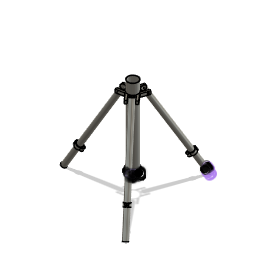
OpenTripod (Autodesk Fusion 360 design; units mm, degrees)
Autodesk Fusion 360 part; units mm, degrees
sketch "Sketch4" plane through (0, 0, 0) normal (0, 1, 0) x (1, 0, 0)
  circle A0 centre (0, 0) radius 25
  circle A1 centre (0, 0) radius 23
  dimension "d26" = 50
  dimension "d27" = 46
  constraint coincident A0.centre A1.centre
  constraint concentric A0 A1
  measures "d26" diameter of A0
  measures "d27" diameter of A1
extrude "Extrude6" add sketch "Sketch4" along normal blind 1000 makes body 1
sketch "Sketch1" plane through (0, 0, 0) normal (0, 1, 0) x (1, 0, 0)
  circle A0 centre (0, 0) radius 50
  circle A1 centre (0, 0) radius 47.5
  dimension "d1" = 100
  dimension "d2" = 95
  constraint coincident A0.centre A1.centre
  constraint concentric A0 A1
  measures "d1" diameter of A0
  measures "d2" diameter of A1
extrude "Extrude1" add sketch "Sketch1" along normal blind 800 separate body makes body 2
sketch "Sketch2" plane through (0, 800, 0) normal (0, 1, 0) x (-1, 0, 0)
  circle A0 centre (0, 0) radius 47.5
  circle A1 centre (0, 0) radius 50
  circle A2 centre (0, 0) radius 51
  circle A3 centre (0, 0) radius 60
  line L0 (0, 0) -> (-51, 0) construction
  line L1 (-51, 0) -> (-60, 0)
  line L2 (0, 0) -> (59.0885, 10.4189) construction
  line L3 (0, 0) -> (60, 0) construction
  line L4 (59.0885, 10.4189) -> (93.5567, 16.4966) construction
  circle A4 centre (93.5567, 16.4966) radius 25
  line L5 (93.5567, 16.4966) -> (89.2155, 41.1168) construction
  line L6 (89.2155, 41.1168) -> (88.3473, 46.0408) construction
  line L7 (88.3473, 46.0408) -> (45.9627, 38.5673)
  line L8 (88.3473, 46.0408) -> (108.0434, 49.5138)
  line L9 (108.0434, 49.5138) -> (104.5705, 69.2099)
  line L10 (104.5705, 69.2099) -> (23.98, 54.9996)
  line L11 (98.7662, -13.0477) -> (56.3816, -20.5212)
  line L12 (121.9353, -29.2708) -> (41.3448, -43.4811)
  line L13 (98.7662, -13.0477) -> (118.4623, -9.5747)
  line L14 (118.4623, -9.5747) -> (121.9353, -29.2708)
  line L15 (-38.0835, 92.0579) -> (-10.4189, 59.0885)
  line L16 (-38.0835, 92.0579) -> (-50.9392, 107.3787)
  line L17 (-50.9392, 107.3787) -> (-35.6184, 120.2345)
  line L18 (-35.6184, 120.2345) -> (16.9834, 57.5462)
  line L19 (-84.0462, 53.4906) -> (-56.3816, 20.5212)
  line L20 (-84.0462, 53.4906) -> (-96.9019, 68.8115)
  line L21 (-96.9019, 68.8115) -> (-112.2228, 55.9557)
  line L22 (-112.2228, 55.9557) -> (-59.6211, -6.7326)
  line L23 (-60.6827, -79.0102) -> (-45.9627, -38.5673)
  line L24 (-60.6827, -79.0102) -> (-67.5231, -97.804)
  line L25 (-67.5231, -97.804) -> (-86.3169, -90.9636)
  line L26 (-86.3169, -90.9636) -> (-58.3282, -14.0651)
  line L27 (-4.3011, -99.5314) -> (10.4189, -59.0885)
  line L28 (-4.3011, -99.5314) -> (-11.1415, -118.3253)
  line L29 (-11.1415, -118.3253) -> (7.6523, -125.1657)
  line L30 (7.6523, -125.1657) -> (35.6411, -48.2671)
  dimension "d7" = 102
  dimension "d8" = 120
  dimension "d24" = 10
  dimension "d30" = 35
  dimension "d31" = 50
  dimension "d32" = 5
  dimension "d33" = 20
  dimension "d34" = 20
  dimension "d36" = 360
  constraint coincident A0.centre A1.centre
  constraint concentric A2 A3
  constraint coincident A2 L0.end
  constraint horizontal L0
  constraint coincident A3 L1.end
  constraint parallel L0 L1
  constraint horizontal L3
  constraint coincident A3 L2.end
  constraint parallel L2 L4
  constraint coincident L4.end A4.centre
  constraint coincident A4 L5.end
  constraint perpendicular L4 L5
  constraint parallel L5 L6
  constraint coincident A3 L7.end
  constraint parallel L4 L7
  constraint perpendicular L6 L8
  constraint perpendicular L8 L9
  constraint coincident A3 L10.end
  constraint perpendicular L9 L10
  constraint symmetric L4 L6.end L11.start
  constraint symmetric L4 L7.end L11.end
  constraint symmetric L4 L8.end L13.end
  constraint symmetric L4 L9.end L12.start
  constraint symmetric L4 L10.end L12.end
  measures "d7" diameter of A2
  measures "d8" diameter of A3
  measures "d24" angle of L2 L3
  measures "d30" distance of L2.end L4.end
  measures "d31" diameter of A4
  measures "d32" distance of L5.end L6.end
  measures "d33" distance of L6.end L8.end
  measures "d34" distance of L8.end L9.end
extrude "Extrude2" add sketch "Sketch2" against normal blind 30 separate body contours A3 | A3 L7 L8 L9 L10 | A3 L11 L12 L13 L14 | A3 L15 L16 L17 L18 | A3 L27 L28 L29 L30 | A3 L19 L20 L21 L22 | A3 L23 L24 L25 L26 makes body 3
sketch "Sketch5" plane through (-8.6824, 0, -49.2404) normal (-0.173648, 0, -0.984808) x (-0.984808, 0, 0.173648)
  line L0 (115, 800) -> (33.1662, 800)
  line L1 (33.1662, 800) -> (33.1662, 770)
  line L2 (33.1662, 770) -> (115, 770)
  line L3 (115, 770) -> (115, 800)
  line L4 (115, 800) -> (80, 770) construction
  circle A0 centre (94.9882, 782.8471) radius 4.1
  dimension "d37" = 8.2
  constraint coincident L0.start L3.end
  constraint coincident L2 L4.end
  constraint coincident L4 A0.centre
  measures "d37" diameter of A0
extrude "Extrude7" cut sketch "Sketch5" against normal blind 100 contours A0 bodies 3
pattern_circular "C-Pattern1" count 3 over 360 about axis through (0, 800, 0) along (0, -1, 0) of "Extrude7"
ref_plane "WorkPlane1" through (28.5521, 785, -78.4463) normal (-0.939693, 0, -0.34202) x (0.34202, 0, -0.939693)
sketch "Sketch6" plane through (0, 0, 0) normal (-0.939693, 0, -0.34202) x (0.34202, 0, -0.939693)
  circle A0 centre (94.9882, -782.8471) radius 4.1
move_body "Move1" bodies 1 to x (1, 0, 0) y (0, 1, 0) z (0, 0, 1) at (32.4879, -217.1529, -89.2597)
move_body "Move2" bodies 1 to x (1, 0, 0) y (0, 1, 0) z (0, 0, 1) at (0, 25, 0)
move_body "Move3" bodies 1 to x (0.984328, 0.17101, 0.043059) y (-0.17101, 0.866025, 0.469846) z (0.043059, -0.469846, 0.881697) at (138.2273, 57.3875, -379.7763)
pattern_circular "C-Pattern2" count 3 over 360 about axis through (0, 1.75, 0) along (0, 1, 0) of bodies 1 makes body 4 at (-251.7543, 521.8007, 66.6853) makes body 5 at (148.9374, 521.2461, 212.5381)
move_body "Move4" bodies 2 to x (1, 0, 0) y (0, 1, 0) z (0, 0, 1) at (0, 100, 0)
sketch "Sketch7" plane through (0, 100, 0) normal (0, -1, 0) x (1, 0, 0)
  circle A0 centre (0, 0) radius 47.5
  circle A1 centre (0, 0) radius 50
  circle A2 centre (0, 0) radius 50
  circle A3 centre (0, 0) radius 51
  circle A4 centre (0, 0) radius 60
  line L0 (0, 0) -> (60, 0)
  line L1 (0, 0) -> (59.0885, -10.4189)
  line L2 (0, 0) -> (-59.7717, 5.2293) construction
  line L3 (0, 0) -> (60, 0) construction
  arc A5 (-57.391, 17.5006) -> (-59.5581, -7.2688) centre (-59.7717, 5.2293) ccw
  arc A6 (-55.7204, 22.2539) -> (-58.7382, -12.2401) centre (-59.7717, 5.2293) ccw
  arc A7 (13.5396, -58.4524) -> (36.074, -47.9444) centre (25.3571, -54.3785) ccw
  arc A8 (8.5877, -59.3822) -> (39.9694, -44.7487) centre (25.3571, -54.3785) ccw
  arc A9 (43.8514, 40.9518) -> (23.484, 55.2132) centre (34.4146, 49.1491) ccw
  arc A10 (47.1327, 37.1283) -> (18.7689, 56.9889) centre (34.4146, 49.1491) ccw
  line L4 (60, 0) -> (70, 0)
  line L5 (59.0885, -10.4189) -> (68.9365, -12.1554)
  line L6 (68.9365, -12.1554) -> (67.2001, -22.0034)
  line L7 (67.2001, -22.0034) -> (56.5255, -20.1212)
  line L8 (70, 0) -> (70, 10)
  line L9 (70, 10) -> (59.1608, 10)
  dimension "d51" = 1
  dimension "d52" = 10
  dimension "d53" = 170
  dimension "d56" = 175
  dimension "d57" = 25
  dimension "d58" = 35
  dimension "d60" = 360
  dimension "d65" = 10
  dimension "d66" = 10
  dimension "d67" = 10
  constraint coincident A0.centre A1.centre
  constraint coincident A4 L0.end
  constraint horizontal L0
  constraint coincident A4 L1.end
  constraint horizontal L3
  constraint coincident A4 L2.end
  constraint coincident L2.end A5.centre
  constraint coincident A4 A5.end
  constraint coincident A4 A6.end
  constraint coincident A4 A5.start
  constraint coincident A4 A6.start
  constraint parallel L0 L4
  constraint parallel L1 L5
  constraint perpendicular L5 L6
  constraint coincident A4 L7.end
  constraint perpendicular L6 L7
  constraint perpendicular L4 L8
  constraint coincident A4 L9.end
  constraint perpendicular L8 L9
  measures "d53" angle of L0 L1
  measures "d56" angle of L2 L3
  measures "d57" diameter of A5
  measures "d58" diameter of A6
  measures "d65" distance of L1.end L5.end
  measures "d66" distance of L5.end L6.end
  measures "d67" distance of L4.end L8.end
extrude "Extrude8" add sketch "Sketch7" against normal blind 50 separate body contours A3 A4 L0 L1 | A4 L4 L8 L9 | A4 L5 L6 L7 picked at (-51.1928, 24.8494) makes body 6
extrude "Extrude9" add sketch "Sketch7" against normal blind 15 contours A4 A9 A10 | A4 A7 A8 | A4 A5 A6 bodies 6
fillet "Fillet1" radius 3 6 edges at (41.5843, 115, 59.3885) (30.6398, 100, -65.7073) (-72.2241, 100, 6.3188) (41.5843, 100, 59.3885) (-72.2241, 115, 6.3188) (30.6398, 115, -65.7073) on bodies 6
sketch "Sketch8" plane through (-1.7365, 0, -9.8481) normal (-0.173648, 0, -0.984808) x (-0.984808, 0, 0.173648)
  line L0 (-70, 100) -> (-59.1608, 100)
  line L1 (-59.1608, 100) -> (-59.1608, 150)
  line L2 (-59.1608, 150) -> (-70, 150)
  line L3 (-70, 150) -> (-70, 100)
  line L4 (-59.1608, 125) -> (-70, 125) construction
  line L5 (-70, 100) -> (-59.1608, 110.8392) construction
  line L6 (-70, 100) -> (-55.1379, 100) construction
  circle A0 centre (-64.5804, 105.4196) radius 3.7
  circle A1 centre (-64.5804, 105.4196) radius 2.1
  circle A2 centre (-64.5804, 144.5804) radius 2.1
  circle A3 centre (-64.5804, 144.5804) radius 3.7
  dimension "d68" = 45
  dimension "d69" = 7.4
  dimension "d70" = 4.2
  constraint midpoint L1 L4.start
  constraint midpoint L3 L4.end
  constraint horizontal L6
  constraint coincident L0.start L3.end
  constraint coincident L1 L5.end
  constraint midpoint L5 A0.centre
  constraint concentric A0 A1
  constraint symmetric L4 A0 A3
  constraint symmetric L4 A1 A2
  measures "d68" angle of L5 L6
  measures "d69" diameter of A0
  measures "d70" diameter of A1
extrude "Extrude10" cut sketch "Sketch8" against normal blind 4.2 contours A0 | A1 | A2 | A3 bodies 6
extrude "Extrude11" cut sketch "Sketch8" against normal up to surface (10 mm away) contours A1 | A2 bodies 6
sketch "Sketch9" plane through (0, 0, 10) normal (0, 0, 1) x (1, 0, 0)
  line L0 (59.1608, 100) -> (70, 100)
  line L1 (70, 100) -> (70, 150)
  line L2 (70, 150) -> (59.1608, 150)
  line L3 (59.1608, 150) -> (59.1608, 100)
  line L4 (59.1608, 125) -> (70, 125) construction
  line L5 (70, 150) -> (59.1608, 139.1608) construction
  line L6 (70, 150) -> (85.3289, 150) construction
  line L7 (68.7804, 147.0053) -> (64.5804, 149.4301)
  line L8 (64.5804, 149.4301) -> (60.3804, 147.0053)
  line L9 (60.3804, 147.0053) -> (60.3804, 142.1555)
  line L10 (60.3804, 142.1555) -> (64.5804, 139.7307)
  line L11 (64.5804, 139.7307) -> (68.7804, 142.1555)
  line L12 (68.7804, 142.1555) -> (68.7804, 147.0053)
  circle A0 centre (64.5804, 144.5804) radius 2.1
  circle A1 centre (64.5804, 105.4196) radius 2.1
  line L13 (68.7804, 107.8445) -> (68.7804, 102.9947)
  line L14 (68.7804, 102.9947) -> (64.5804, 100.5699)
  line L15 (64.5804, 100.5699) -> (60.3804, 102.9947)
  line L16 (60.3804, 102.9947) -> (60.3804, 107.8445)
  line L17 (60.3804, 107.8445) -> (64.5804, 110.2693)
  line L18 (64.5804, 110.2693) -> (68.7804, 107.8445)
  point P0 (64.5804, 144.5804)
  dimension "d75" = 135
  dimension "d76" = 4.2
  dimension "d77" = 4.2
  constraint midpoint L3 L4.start
  constraint midpoint L1 L4.end
  constraint horizontal L6
  constraint coincident L1.end L2.start
  constraint coincident L3 L5.end
  constraint midpoint L5 P0
  constraint coincident P0 A0.centre
  constraint vertical L12
  constraint symmetric L4 L7.start L13.end
  constraint symmetric L4 L7.end L14.end
  constraint symmetric L4 L8.end L15.end
  constraint symmetric L4 L9.end L16.end
  constraint symmetric L4 L10.end L17.end
  constraint symmetric L4 L11.end L13.start
  constraint symmetric L4 A0 A1
  measures "d75" angle of L5 L6
  measures "d76" distance of P0 L12
  measures "d77" diameter of A0
extrude "Extrude12" cut sketch "Sketch9" against normal blind 4.2 contours L7 L8 L9 L10 L11 L12 | A0 | A1 | L13 L14 L15 L16 L17 L18 bodies 6
extrude "Extrude13" cut sketch "Sketch9" against normal up to surface (10 mm away) contours A0 | A1 bodies 6
fillet "Fillet2" radius 2 2 edges at (51, 125, 0) (50.2252, 125, -8.8561) on bodies 6
fillet "Fillet3" radius 1 2 edges at (56.5255, 125, -20.1212) (59.1608, 125, 10) on bodies 6
fillet "Fillet4" radius 1 4 edges at (68.9365, 125, -12.1554) (67.2001, 125, -22.0034) (70, 125, 0) (70, 125, 10) on bodies 6
sketch "Sketch10" plane through (58.9179, -298.3706, -161.8755) normal (0.17101, -0.866025, -0.469846) x (-0.939693, 0, -0.34202)
  circle A0 centre (0, 473.6858) radius 23
  circle A1 centre (0, 473.6858) radius 25
  circle A2 centre (0, 473.6858) radius 26
  circle A3 centre (0, 473.6858) radius 31
  line L0 (0, 473.6858) -> (31, 473.6858)
  line L1 (0, 473.6858) -> (30.529, 479.0689)
  line L2 (0, 473.6858) -> (-30.882, 470.9839) construction
  line L3 (31, 473.6858) -> (36, 473.6858)
  line L4 (36, 473.6858) -> (36, 463.6858)
  line L5 (36, 463.6858) -> (29.3428, 463.6858)
  line L6 (30.529, 479.0689) -> (35.4531, 479.9371)
  line L7 (35.4531, 479.9371) -> (33.7166, 489.7852)
  line L8 (33.7166, 489.7852) -> (27.1605, 488.6292)
  arc A4 (-29.4385, 483.4003) -> (-27.3044, 459.0069) centre (-30.882, 470.9839) ccw
  arc A5 (-22.8966, 461.3672) -> (-22.1313, 462.0579) centre (-30.882, 470.9839) ccw
  arc A6 (-27.4245, 488.139) -> (-24.4981, 454.6899) centre (-30.882, 470.9839) ccw
  arc A7 (-21.7919, 485.9378) -> (-22.6609, 486.4327) centre (-30.882, 470.9839) ccw
  dimension "d88" = 1
  dimension "d89" = 6
  dimension "d92" = 170
  dimension "d93" = 5
  dimension "d94" = 10
  dimension "d95" = 5
  dimension "d96" = 10
  dimension "d118" = 25
  dimension "d119" = 35
  constraint coincident A0.centre A1.centre
  constraint coincident A3 L0.end
  constraint horizontal L0
  constraint coincident A3 L1.end
  constraint coincident A3 L2.end
  constraint parallel L0 L3
  constraint perpendicular L0 L4
  constraint coincident A3 L5.end
  constraint perpendicular L4 L5
  constraint parallel L1 L6
  constraint perpendicular L6 L7
  constraint coincident A3 L8.end
  constraint perpendicular L7 L8
  constraint coincident L2.end A4.centre
  constraint concentric A4 A6
  constraint coincident A3 A4.start
  constraint coincident A1 A5.end
  constraint coincident A3 A4.end
  constraint coincident A2 A5.start
  constraint concentric A4 A5
  constraint coincident A2 A7.end
  constraint coincident A3 A6.start
  constraint coincident A1 A7.start
  constraint concentric A6 A7
  constraint coincident A3 A6.end
  measures "d92" angle of L0 L1
  measures "d93" angle of L1 L2
  measures "d94" distance of L3.end L4.end
  measures "d95" distance of L1.end L6.end
  measures "d96" distance of L6.end L7.end
  measures "d118" diameter of A4
  measures "d119" diameter of A6
extrude "Extrude14" add sketch "Sketch10" against normal blind 30 separate body contours A2 A3 L0 L1 | A3 L3 L4 L5 | A3 L6 L7 L8 | A3 A4 A6 picked at (24.4161, 489.8407) makes body 7
fillet "Fillet5" radius 3 2 edges at (238.8208, -63.4233, -529.4533) (233.6905, -37.4426, -515.3579) on bodies 7
sketch "Sketch11" plane through (216.7427, 234.6252, -353.5757) normal (0.454874, 0.492404, -0.742043) x (-0.852564, 0, -0.522623)
  line L0 (145.4095, -331.6777) -> (152.0335, -331.0136)
  line L1 (152.0335, -331.0136) -> (149.0409, -301.1632)
  line L2 (149.0409, -301.1632) -> (142.4169, -301.8273)
  line L3 (142.4169, -301.8273) -> (145.4095, -331.6777)
  line L4 (137.1007, -302.3603) -> (140.0934, -332.2106)
  line L5 (92.3328, -336.9989) -> (89.3401, -307.1486)
  line L6 (149.0409, -301.1632) -> (138.0796, -312.1244) construction
  line L7 (149.0409, -301.1632) -> (164.5424, -301.1632) construction
  circle A0 centre (143.5602, -306.6438) radius 1.6
  circle A1 centre (143.5602, -306.6438) radius 2.85
  line L8 (150.5372, -316.0884) -> (143.9132, -316.7525) construction
  circle A2 centre (143.5602, -306.6438) radius 3.5
  circle A3 centre (145.574, -326.73) radius 1.6
  circle A4 centre (145.574, -326.73) radius 2.85
  circle A5 centre (145.574, -326.73) radius 3.5
  line L9 (145.4095, -331.6777) -> (142.4169, -301.8273)
  dimension "d97" = 135
  dimension "d98" = 3.2
  dimension "d99" = 5.7
  dimension "d100" = 7
  constraint horizontal L7
  constraint coincident L1.end L2.start
  constraint coincident L4 L6.end
  constraint midpoint L6 A0.centre
  constraint concentric A0 A1
  constraint midpoint L1 L8.start
  constraint midpoint L3 L8.end
  constraint concentric A0 A2
  constraint symmetric A0 L8 A3
  constraint symmetric A1 L8 A4
  constraint symmetric L8 A2 A5
  measures "d97" angle of L6 L7
  measures "d98" diameter of A0
  measures "d99" diameter of A1
  measures "d100" diameter of A2
extrude "Extrude15" cut sketch "Sketch11" along normal blind 26.5 contours L3 A4 A5 L9 | L3 A4 A5 L9 | L3 A3 A4 L9 | L3 A3 A4 L9 | L3 A3 L9 | L3 A3 L9 | L3 A1 A2 L9 | L3 A1 A2 L9 | L3 A0 A1 L9 | L3 A0 A1 L9 | L3 A0 L9 | L3 A0 L9 bodies 7
extrude "Extrude16" cut sketch "Sketch11" against normal blind 3.2 contours L3 A3 A4 L9 | L3 A3 A4 L9 | L3 A3 L9 | L3 A3 L9 | L3 A0 A1 L9 | L3 A0 A1 L9 | L3 A0 L9 | L3 A0 L9 bodies 7
extrude "Extrude17" cut sketch "Sketch11" against normal up to surface (10 mm away) contours L3 A3 L9 | L3 A3 L9 | L3 A0 L9 | L3 A0 L9 bodies 7
sketch "Sketch12" plane through (137.3429, 231.8429, -377.3464) normal (-0.296198, -0.5, 0.813798) x (0.939693, 0, 0.34202)
  line L0 (-36, -344.5287) -> (-29.3428, -344.5287)
  line L1 (-29.3428, -344.5287) -> (-29.3428, -314.5287)
  line L2 (-29.3428, -314.5287) -> (-36, -314.5287)
  line L3 (-36, -314.5287) -> (-36, -344.5287)
  line L4 (-36, -329.5287) -> (-29.3428, -329.5287) construction
  line L5 (24, -314.5287) -> (24, -344.5287) construction
  line L6 (-24, -344.5287) -> (-24, -314.5287) construction
  line L7 (-24, -314.5287) -> (-36, -326.5287) construction
  line L8 (-24, -314.5287) -> (-7.0294, -314.5287) construction
  line L9 (-33.2, -322.3762) -> (-30, -324.2237)
  line L10 (-30, -324.2237) -> (-26.8, -322.3762)
  line L11 (-26.8, -322.3762) -> (-26.8, -318.6812)
  line L12 (-26.8, -318.6812) -> (-30, -316.8336)
  line L13 (-30, -316.8336) -> (-33.2, -318.6812)
  line L14 (-33.2, -318.6812) -> (-33.2, -322.3762)
  circle A0 centre (-30, -320.5287) radius 4
  circle A1 centre (-30, -320.5287) radius 1.6
  line L15 (-33.2, -336.6812) -> (-30, -334.8336)
  line L16 (-33.2, -340.3762) -> (-33.2, -336.6812)
  line L17 (-30, -334.8336) -> (-26.8, -336.6812)
  line L18 (-26.8, -336.6812) -> (-26.8, -340.3762)
  line L19 (-26.8, -340.3762) -> (-30, -342.2237)
  line L20 (-30, -342.2237) -> (-33.2, -340.3762)
  circle A2 centre (-30, -338.5287) radius 1.6
  circle A3 centre (-30, -338.5287) radius 4
  point P0 (-30, -320.5287)
  dimension "d107" = 135
  dimension "d108" = 3.2
  dimension "d109" = 8
  dimension "d110" = 3.2
  constraint midpoint L3 L4.start
  constraint midpoint L1 L4.end
  constraint horizontal L8
  constraint coincident L6.end L7.start
  constraint coincident L3 L7.end
  constraint midpoint L7 P0
  constraint vertical L14
  constraint coincident P0 A0.centre
  constraint concentric A0 A1
  constraint symmetric L4 L9.start L15.start
  constraint symmetric L4 L9.end L15.end
  constraint symmetric L4 L10.end L17.end
  constraint symmetric L4 L11.end L18.end
  constraint symmetric L4 L12.end L19.end
  constraint symmetric L4 L13.end L16.start
  constraint symmetric L4 A0 A3
  constraint symmetric L4 A1 A2
  measures "d107" angle of L7 L8
  measures "d108" distance of P0 L14
  measures "d109" diameter of A0
  measures "d110" diameter of A1
extrude "Extrude18" cut sketch "Sketch12" along normal blind 58 contours L1 L15 L16 L17 L19 L20 A3 | L1 L17 L18 L19 A3 | L1 L15 L16 L17 L19 L20 A2 | L1 L17 L18 L19 A2 | L1 L10 L11 L12 A0 | L1 L9 L10 L12 L13 L14 A0 | L1 A2 | L1 A2 | L1 L10 L11 L12 A1 | L1 L9 L10 L12 L13 L14 A1 | L1 A1 | L1 A1 bodies 7
extrude "Extrude19" cut sketch "Sketch12" against normal blind 3.2 contours L1 L15 L16 L17 L19 L20 A2 | L1 L17 L18 L19 A2 | L1 A2 | L1 A2 | L1 L10 L11 L12 A1 | L1 L9 L10 L12 L13 L14 A1 | L1 A1 | L1 A1 bodies 7
extrude "Extrude20" cut sketch "Sketch12" against normal up to surface (10 mm away) contours L1 A2 | L1 A2 | L1 A1 | L1 A1 bodies 7
move_body "Move5" bodies 7 to x (0.113851, -0.60325, 0.789384) y (0.332867, 0.771789, 0.541795) z (-0.936076, 0.201076, 0.288671) at (-315.3487, 216.2007, -513.2808)
move_body "Move6" bodies 7 to x (1, 0, 0) y (0, 1, 0) z (0, 0, 1) at (-41.0424, 207.8461, 112.7631)
pattern_circular "C-Pattern3" count 3 over 360 about axis through (0, 100, 0) along (0, 1, 0) of bodies 7 makes body 8 at (-440.5817, 151.7032, 103.2358) makes body 9 at (271.6209, 152.3318, 363.3068)
move_body "Move7" bodies 6 to x (0.996195, 0, -0.087156) y (0, 1, 0) z (0.087156, 0, 0.996195) at (0, 0, 0)
extrude "Extrude21" cut sketch "Sketch6" along normal up to surface (50 mm away) and the other way up to surface (50 mm away) bodies 1
sketch "Sketch13" plane through (46.9846, 0, 17.101) normal (0.939693, 0, 0.34202) x (0.34202, 0, -0.939693)
  circle A0 centre (94.9882, 782.8471) radius 4.1
  line L0 (115, 800) -> (33.1662, 800)
  line L1 (33.1662, 800) -> (33.1662, 770)
  line L2 (33.1662, 770) -> (115, 770)
  line L3 (115, 770) -> (115, 800)
  line L4 (101.9882, 786.8885) -> (94.9882, 790.93)
  line L5 (94.9882, 790.93) -> (87.9882, 786.8885)
  line L6 (87.9882, 786.8885) -> (87.9882, 778.8056)
  line L7 (87.9882, 778.8056) -> (94.9882, 774.7642)
  line L8 (94.9882, 774.7642) -> (101.9882, 778.8056)
  line L9 (101.9882, 778.8056) -> (101.9882, 786.8885)
  point P0 (94.9882, 782.8471)
  dimension "d129" = 7
  constraint coincident P0 A0.centre
  measures "d129" distance of P0 L9
extrude "Extrude22" cut sketch "Sketch13" against normal blind 7 contours L4 L5 L6 L7 L8 L9 bodies 3
pattern_circular "C-Pattern4" count 3 over 360 about axis through (0, 100, 0) along (0, 1, 0) of "Extrude22"
equation "Tolerance = 0.2 mm"
equation "CenterPoleSize = 100 mm"
equation "d7 = CenterPoleSize + 2 mm"
equation "LegDiameter = 50 mm"
equation "d26 = LegDiameter"
equation "d27 = LegDiameter - 4 mm"
equation "d30 = LegDiameter / 2 + 10 mm"
equation "d31 = LegDiameter"
equation "d37 = 8 mm + Tolerance"
equation "d43 = LegDiameter / 2"
equation "d69 = 7.2 mm + Tolerance"
equation "d70 = 4 mm + Tolerance"
equation "d71 = -4 mm - Tolerance"
equation "d76 = 4 mm + Tolerance"
equation "d77 = 4 mm + Tolerance"
equation "d78 = -4 mm - Tolerance"
equation "d98 = 3 mm + Tolerance"
equation "d99 = 5.5 mm + Tolerance"
equation "d103 = -3 mm - Tolerance"
equation "d108 = 3 mm + Tolerance"
equation "d110 = 3 mm + Tolerance"
equation "d113 = -3 mm - Tolerance"
